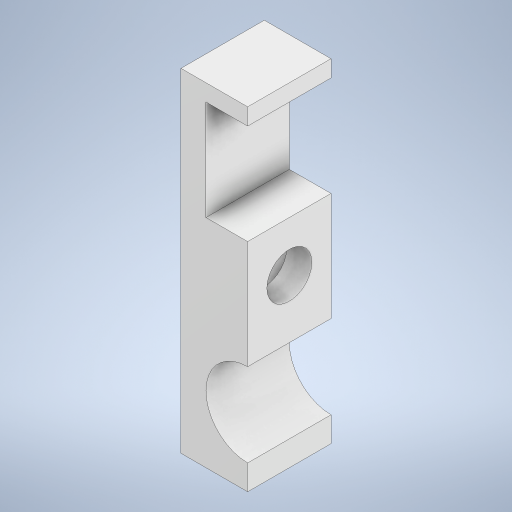
# Autodesk Inventor part: POMSliderAxis
Saved by Autodesk Inventor 2023 (Build 270158000, 158)
## iProperties
Created: 2023-03-28
Part Number: POMSliderAxis
Material: Acetal Resin, White
Document SubType Name: Modeling
Designer: Nathann
Density: 1.425 g/cm^3
Appearance: Smooth - White
Mass: 0.313758 g
Surface Area: 4.29392 cm^2
Volume: 0.220181 cm^3
Author: Nathann
Autodesk Inventor part; units mm, degrees
ref_plane "YZ Plane" through (0, 0, 0) normal (1, 0, 0) x (0, 1, 0)
ref_plane "XZ Plane" through (0, 0, 0) normal (0, 1, 0) x (-1, 0, 0)
ref_plane "XY Plane" through (0, 0, 0) normal (0, 0, 1) x (1, 0, 0)
sketch "Sketch1" plane through (0, 0, 0) normal (0, 0, 1) x (1, 0, 0)
  line L0 (0, 0) -> (4, 0)
  line L1 (4, 0) -> (4, -20)
  line L2 (4, -20) -> (0, -20)
  line L3 (0, -20) -> (0, 0)
  circle A0 centre (4, -4) radius 2.5
  circle A1 centre (4, -16) radius 2.5
  line L4 (1.5, -4) -> (1.5, -7)
  line L5 (1.5, -7) -> (1.5, -1)
  line L6 (4, -7) -> (1.5, -7)
  line L7 (1.5, -1) -> (4, -1)
  point P0 (4, -18.5)
  point P1 (4, -13.5)
  dimension "d2" = 5
  dimension "d0" = 20
  dimension "d1" = 4
  dimension "d3" = 5
  dimension "d4" = 4
  dimension "d5" = 4
  dimension "d6" = 3
  dimension "d7" = 3
  constraints: 16 end point, 5 point on line, 2 parallel, 2 perpendicular, 2 vertical, 1 centre point, 1 horizontal, 1 horizontal alignment, 2 other
  measures "d0" distance between parallel lines of L0 L2
  measures "d1" distance of L0.start L0.end
  measures "d3" diameter of A1
  measures "d4" distance from line of A1.centre L2
  measures "d5" distance from line of L0 point (4, -4)
  measures "d6" distance from line of L7 point (4, -4)
  measures "d7" distance from line of L6 point (4, -4)
extrude "Extrusion1" add sketch "Sketch1" along normal blind 5 contours L0 L1 L7 L5 L4 L6 A1 L2 L3
sketch "Sketch3" plane through (0, -20, 0) normal (-1, 0, 0) x (0, 0, 1)
  circle A0 centre (2.5, 10) radius 1.35
  line L0 (0, 0) -> (5, 0) projected
  line L1 (0, 20) -> (0, 0) projected
  dimension "d10" = 10
  dimension "d11" = 2.5
  dimension "d12" = 20
  dimension "d13" = 2.7
  constraints: 1 centre point
  measures "d10" distance from line of A0.centre L0
  measures "d11" distance from line of L1 A0.centre
  measures "d12" distance of L1.start L0.start
  measures "d13" diameter of A0
extrude "Extrusion2" cut sketch "Sketch3" against normal blind 20
sketch "Sketch4" plane through (0, -20, 0) normal (-1, 0, 0) x (0, 0, 1)
  circle A0 centre (2.5, 10) radius 1.35 projected
  circle A1 centre (2.5, 10) radius 2.45
  point P0 (0, 20)
  dimension "d16" = 4.9
  constraints: 1 centre point, 1 coincident
  measures "d16" diameter of A1
extrude "Extrusion3" cut sketch "Sketch4" against normal blind 2.5 contours A0 | A1
equation "\"d1\" = d4"
equation "\"d5\" = d4"
body "Solid1"
